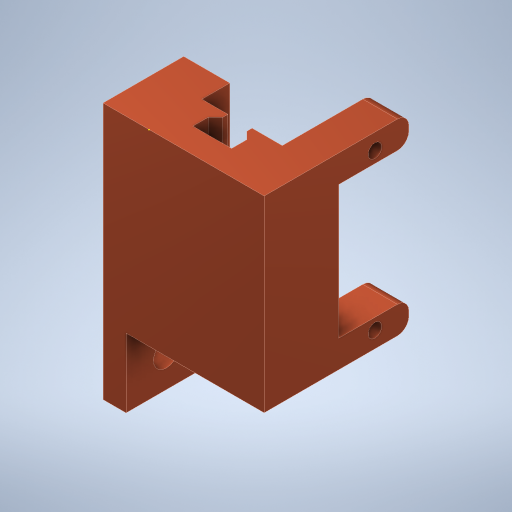
# Autodesk Inventor part: Motor_holder
Saved by Autodesk Inventor 2024.2 (Build 282272000, 272)
## iProperties
Created: 2025-06-02
Part Number: Motor_holder
Material: Měď
Document SubType Name: Modeling
Designer: Elite
Density: 8.94 g/cm^3
Appearance: Měď – satén
Mass: 95.1556 g
Surface Area: 50.1955 cm^2
Volume: 10.6438 cm^3
Author: Elite
Autodesk Inventor part; units mm, degrees
ref_plane "YZ Plane" through (0, 0, 0) normal (1, 0, 0) x (0, 1, 0)
ref_plane "XZ Plane" through (0, 0, 0) normal (0, 1, 0) x (-1, 0, 0)
ref_plane "XY Plane" through (0, 0, 0) normal (0, 0, 1) x (1, 0, 0)
sketch "Náčrt1" plane through (0, 0, 0) normal (0, 0, 1) x (1, 0, 0)
  line L0 (13.97, 23.865) -> (13.97, 9.144)
  line L1 (0, 9.144) -> (0, 0)
  line L2 (4.5409, 9.144) -> (0, 9.144)
  line L3 (4.5409, 8.255) -> (4.5409, 9.144)
  line L4 (3.2709, 6.985) -> (4.5409, 8.255)
  line L5 (3.2709, 4.318) -> (3.2709, 6.985)
  line L6 (8.7319, 9.144) -> (8.7319, 8.255)
  line L7 (13.97, 9.144) -> (8.7319, 9.144)
  line L8 (8.7319, 8.255) -> (10.0019, 6.985)
  line L9 (10.0019, 6.985) -> (10.0019, 4.318)
  line L10 (10.0019, 4.318) -> (3.2709, 4.318)
  line L11 (0, 0) -> (19.97, 0)
  line L12 (13.97, 22.5956) -> (13.97, 25.1349)
  line L13 (13.97, 20.4353) -> (13.97, 18.035)
  line L14 (13.97, 25.1349) -> (19.97, 25.1349)
  line L15 (19.97, 25.1349) -> (19.97, 0)
  constraints: 32 end point, 1 horizontal, 1 vertical
extrude "Vysunutí1" add sketch "Náčrt1" against normal blind 32.6
sketch "Náčrt2" plane through (19.97, 0, 0) normal (1, 0, 0) x (0, 0, -1)
  line L0 (0, 25.1349) -> (32.6, 25.1349) projected
  line L1 (16.3, 25.1349) -> (4.746, 25.1349)
  line L2 (4.746, 25.1349) -> (4.746, 12.9539)
  line L3 (16.3, 25.1349) -> (27.854, 25.1349)
  line L4 (27.854, 25.1349) -> (27.854, 12.9539)
  line L5 (27.854, 12.9539) -> (4.746, 12.9539)
  circle A0 centre (2.8, 19.2349) radius 1.2
  line L6 (16.3, 25.1349) -> (16.3, 15.9225)
  circle A1 centre (29.8, 19.2349) radius 1.2
  point P0 (0, 0)
  point P1 (4.746, 19.0444)
  dimension "d2" = 11.554
  dimension "d3" = 12.181
  dimension "d4" = 11.554
  dimension "d7" = 2.4
  dimension "d8" = 5.9
  dimension "d9" = 1.946
  constraints: 12 end point, 3 perpendicular, 2 centre point, 2 midpoint, 2 point on line, 1 symmetric about line, 1 vertical, 1 other
  measures "d2" distance of L1.start L1.end
  measures "d3" distance of L1.end L2.end
  measures "d4" distance of L1.start L3.end
  measures "d7" diameter of A0
  measures "d8" distance from line of L0 A0.centre
  measures "d9" horizontal distance of point (4.746, 19.044) A0.centre
extrude "Vysunutí2" cut sketch "Náčrt2" against normal blind 32.6 contours L0 L4 L5 L2
extrude "Vysunutí3" cut sketch "Náčrt2" against normal blind 32.6 contours A0 | A1
fillet "Zaoblení1" radius 2 4 edges at (16.97, 25.1349, 0) (16.97, 25.1349, -4.746) (16.97, 25.1349, -27.854) (16.97, 25.1349, -32.6)
sketch "Náčrt3" plane through (0, 0, 0) normal (0, -1, 0) x (1, 0, 0)
  point P0 (0, 0)
sketch "Náčrt4" plane through (0, 0, 0) normal (0, 0, 1) x (1, 0, 0)
  line L0 (13.97, 23.1349) -> (19.97, 23.1349) projected
  line L1 (13.97, 23.1349) -> (13.97, 9.144) projected
  line L2 (13.97, 9.144) -> (8.7319, 9.144) projected
  line L3 (8.7319, 9.144) -> (8.7319, 8.255) projected
  line L4 (8.7319, 8.255) -> (10.0019, 6.985) projected
  line L5 (10.0019, 6.985) -> (10.0019, 4.318) projected
  line L6 (10.0019, 4.318) -> (3.2709, 4.318) projected
  line L7 (3.2709, 4.318) -> (3.2709, 6.985) projected
  line L8 (3.2709, 6.985) -> (4.5409, 8.255) projected
  line L9 (4.5409, 8.255) -> (4.5409, 9.144) projected
  line L10 (4.5409, 9.144) -> (0, 9.144) projected
  line L11 (0, 9.144) -> (0, 0) projected
  line L12 (0, 0) -> (19.97, 0) projected
  line L13 (19.97, 0) -> (19.97, 23.1349) projected
  line L14 (0, 0) -> (-8, 0)
  line L15 (-8, 0) -> (-8, 14)
  line L16 (-8, 14) -> (0, 14)
  line L17 (0, 14) -> (0, 0)
  dimension "d13" = 14
  dimension "d14" = 8
  constraints: 8 end point, 2 parallel, 1 horizontal, 1 perpendicular
  measures "d13" distance of L14.end L15.end
  measures "d14" distance of L15.end L16.end
extrude "Vysunutí4" add sketch "Náčrt4" along normal blind 12 and the other way blind 32.6 contours L14 L15 L16 L17 L11
sketch "Náčrt5" plane through (0, 0, 0) normal (1, 0, 0) x (0, 0, -1)
  line L0 (0, 9.144) -> (0, 0) projected
  line L1 (0, 9.144) -> (32.6, 9.144) projected
  line L2 (32.6, 14) -> (32.6, 9.144) projected
  line L3 (32.6, 14) -> (-12, 14) projected
  line L4 (-12, 0) -> (-12, 14) projected
  line L5 (0, 0) -> (-12, 0) projected
  circle A0 centre (-6.5, 7) radius 2.25
  line L6 (27.854, 12.9539) -> (4.746, 12.9539) projected
  line L7 (16.3, 12.9539) -> (16.3, -5.3216)
  line L8 (32.6, 9.144) -> (32.6, 0)
  line L9 (44.6, 0) -> (44.6, 14)
  line L10 (32.6, 0) -> (44.6, 0)
  circle A1 centre (39.1, 7) radius 2.25
  line L11 (44.6, 14) -> (32.6, 14)
  line L12 (32.6, 14) -> (32.6, 0)
  dimension "d19" = 4.5
  dimension "d20" = 7
  dimension "d21" = 5.5
  constraints: 12 end point, 5 symmetric about line, 2 centre point, 1 collinear, 1 horizontal, 1 midpoint, 1 vertical, 1 other
  measures "d19" diameter of A0
  measures "d20" distance from line of L5 A0.centre
  measures "d21" distance from line of L4 A0.centre
extrude "Vysunutí5" add sketch "Náčrt5" against normal up to surface (8 mm away) contours L2 L11 L9 L10 L8 | A0
sketch "Náčrt6" plane through (0, 0, 12) normal (0, 0, 1) x (1, 0, 0)
  line L0 (-8, 14) -> (-8, 0) projected
  line L1 (-8, 0) -> (0, 0) projected
  line L2 (0, 0) -> (0, 14) projected
  line L3 (0, 14) -> (-8, 14) projected
  line L4 (0, 14) -> (-4, 14)
  line L5 (-4, 14) -> (-4, 0)
  line L6 (-4, 0) -> (0, 0)
  line L7 (0, 0) -> (0, 14)
  dimension "d24" = 4
  constraints: 8 end point, 2 parallel, 1 horizontal, 1 midpoint, 1 perpendicular
  measures "d24" distance between parallel lines of L5 L2
extrude "Vysunutí6" cut sketch "Náčrt6" against normal blind 12 contours L3 L2 L1 L5
extrude "Vysunutí7" cut sketch "Náčrt5" against normal blind 4 contours L2 L11 L9 L10 L8
sketch "Náčrt7" plane through (0, 0, 12) normal (0, 0, 1) x (1, 0, 0)
  line L0 (-4, 0) -> (-4, 14) projected
  line L1 (-4, 14) -> (-8, 14) projected
  line L2 (-8, 14) -> (-8, 0) projected
  line L3 (-8, 0) -> (-4, 0) projected
  point P0 (0, 0)
extrude "Vysunutí8" cut sketch "Náčrt7" against normal up to surface (12 mm away)
